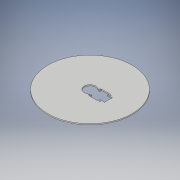
# Autodesk Inventor part: platform 1
Saved by Autodesk Inventor 2019 (Build 230136000, 136)
## iProperties
Created: 2019-02-09
Part Number: platform 1
Material: Generic
Document SubType Name: Modeling
Designer: mashi
Density: 1 g/cm^3
Appearance: Default
Author: mashi
Autodesk Inventor part; units mm, degrees
ref_plane "YZ Plane" through (0, 0, 0) normal (1, 0, 0) x (0, 1, 0)
ref_plane "XZ Plane" through (0, 0, 0) normal (0, 1, 0) x (-1, 0, 0)
ref_plane "XY Plane" through (0, 0, 0) normal (0, 0, 1) x (1, 0, 0)
sketch "Sketch1" plane through (0, 0, 0) normal (0, 1, 0) x (-1, 0, 0)
  circle A0 centre (0, 0) radius 120
  circle A1 centre (-9, 10) radius 1
  circle A2 centre (-9, -10) radius 1
  circle A3 centre (-29, -10) radius 1
  circle A4 centre (-29, 10) radius 1
  arc A5 (-8.0467, -7.5) -> (-8.0467, 7.5) centre (0, 0) ccw
  line L0 (-9, -7.5) -> (-8.0467, -7.5)
  line L1 (-9, -7.5) -> (-11, -7.5)
  line L2 (-11, -7.5) -> (-11, -11.5)
  line L3 (-29, -10) -> (-26, -10)
  line L4 (-11, -11.5) -> (-26, -11.5)
  line L5 (-26, -11.5) -> (-26, -7.5)
  line L6 (-26, -7.5) -> (-35, -7.5)
  line L7 (-35, -7.5) -> (-35, 0)
  line L8 (-9, 7.5) -> (-8.0467, 7.5)
  line L9 (-9, 7.5) -> (-11, 7.5)
  line L10 (-11, 7.5) -> (-11, 11.5)
  line L11 (-11, 11.5) -> (-26, 11.5)
  line L12 (-26, 11.5) -> (-26, 7.5)
  line L13 (-26, 7.5) -> (-35, 7.5)
  line L14 (-35, 7.5) -> (-35, 0)
  dimension "d0" = 240
  dimension "d5" = 2
  dimension "d6" = 2
  dimension "d7" = 2
  dimension "d8" = 2
  dimension "d9" = 22
  dimension "d12" = 2
  dimension "d13" = 3
  dimension "d14" = 4
  dimension "d15" = 9
  constraints: 30 end point, 6 centre point, 4 horizontal, 4 perpendicular, 2 coincident, 2 point on circle
  measures "d0" diameter of A0
  measures "d5" diameter of A1
  measures "d6" diameter of A2
  measures "d7" diameter of A3
  measures "d8" diameter of A4
  measures "d9" diameter of A5
  measures "d12" distance of L0.start L1.end
  measures "d13" distance of L3.start L3.end
  measures "d14" distance of L4.end L5.end
  measures "d15" distance of L5.end L6.end
extrude "Extrusion1" add sketch "Sketch1" along normal blind 2
sketch "Sketch3" plane through (0, 2, 0) normal (0, 1, 0) x (1, 0, 0)
  circle A0 centre (-40, 0) radius 4
  circle A1 centre (40, 0) radius 4
  circle A2 centre (0, -40) radius 4
  circle A3 centre (0, 40) radius 4
  point P0 (0, 0)
  dimension "d22" = 8
  dimension "d23" = 8
  dimension "d24" = 8
  dimension "d25" = 8
  constraints: 4 centre point
  measures "d22" diameter of A0
  measures "d23" diameter of A1
  measures "d24" diameter of A2
  measures "d25" diameter of A3
extrude "Extrusion2" add sketch "Sketch3" along normal blind 12
sketch "Sketch4" plane through (0, 2, 0) normal (0, 1, 0) x (1, 0, 0)
  circle A0 centre (0, 0) radius 60
  circle A1 centre (0, 0) radius 120.1645
  dimension "d28" = 120
  dimension "d29" = 240.329
  constraints: 2 centre point, 2 coincident
  measures "d28" diameter of A0
  measures "d29" diameter of A1
extrude "Extrusion3" cut sketch "Sketch4" against normal blind 12
move faces "Move5" translate (0, -47.625, 0) faces at (-2.1262, 14, 40.6196)
move faces "Move6" translate (0, -71.438, 0) faces at (-41.1806, 14, -0.6196)
move faces "Move7" translate (0, -49.213, 0) faces at (0.7574, 14, -41.0973)
move faces "Move8" translate (0, -36.513, 0) faces at (38.8194, 14, -0.6196)
sketch "Sketch5" plane through (0, 2, 0) normal (0, 1, 0) x (1, 0, 0)
  circle A0 centre (0, 0) radius 28
  line L0 (0, 0) -> (19.799, 19.799)
  line L1 (0, 0) -> (28, 0) construction
  line L2 (19.799, 19.799) -> (-19.799, 19.799)
  line L3 (-19.799, 19.799) -> (-19.799, -19.799)
  line L4 (-19.799, -19.799) -> (19.799, -19.799)
  circle A1 centre (-19.799, -19.799) radius 3
  circle A2 centre (-19.799, 19.799) radius 3
  circle A3 centre (19.799, 19.799) radius 3
  circle A4 centre (19.799, -19.799) radius 3
  line L5 (19.799, 19.799) -> (42.4264, 42.4264)
  circle A5 centre (0, 0) radius 80
  circle A6 centre (0, 0) radius 60
  dimension "d56" = 56
  dimension "d57" = 45
  dimension "d58" = 6
  dimension "d59" = 6
  dimension "d60" = 6
  dimension "d62" = 6
  dimension "d63" = 32
  dimension "d64" = 160
  constraints: 12 end point, 7 centre point, 7 coincident, 4 point on circle, 2 horizontal, 2 point on line, 1 equal length, 1 perpendicular
  measures "d56" diameter of A0
  measures "d57" angle of L1 L0
  measures "d58" diameter of A1
  measures "d59" diameter of A2
  measures "d60" diameter of A3
  measures "d62" diameter of A4
  measures "d63" distance of L5.start L5.end
  measures "d64" diameter of A5
extrude "Extrusion4" add sketch "Sketch5" against normal blind 2 contours A5
body "Solid1"
